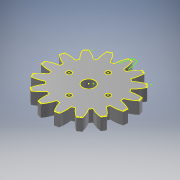
# Autodesk Inventor part: Spur Gear1
Saved by Autodesk Inventor 2017 (Build 210142000, 142)
## iProperties
Created: 2018-10-15
Part Number: Spur Gear1
Material: Steel
Document SubType Name: Modeling
Designer: Tom
Categories: <?xml version="1.0" encoding="UTF-16"?> <MemberInstance><Categories><FamilyTemplate><FamilyTemplateParameter ValueType="xs:double" Id="1" ObjectReferenceKey="da_z" ObjectType="kUserParameterObject"/><FamilyTemplateParameter ValueType="xs:double" Id="2" ObjectReferenceKey="da_b" ObjectType="kUserParameterObject"/><FamilyTemplateParameter ValueType="xs:double" Id="3" ObjectReferenceKey="da_beta" ObjectType="kUserParameterObject"/><FamilyTemplateParameter ValueType="xs:double" Id="4" ObjectReferenceKey="da_da" ObjectType="kUserParameterObject"/><FamilyTemplateParameter ValueType="xs:double" Id="5" ObjectReferenceKey="da_aw" ObjectType="kUserParameterObject"/><FamilyTemplateParameter ValueType="xs:string" Id="6" ObjectReferenceKey="EAIAABAAAACIAQAAAAAAAIAAAAAAAAAA" ObjectType="83910656" SubObjectId="SurfaceGeometry"/></FamilyTemplate><ParamToTemplateMap><ParamToTemplate CategoryParameter="//CategoryParameter[@InternalName='046C89C9-8512-4d59-83FE-43B91F4F132A']" TemplateParameter="1"/><ParamToTemplate CategoryParameter="//CategoryParameter[@InternalName='2552DF32-E462-4b46-AEBF-C6C7768E72AC']" TemplateParameter="2"/><ParamToTemplate CategoryParameter="//CategoryParameter[@InternalName='C9EE641D-15FC-4fae-A226-E94C4372FDD7']" TemplateParameter="3"/><ParamToTemplate><ParamToTemplate CategoryParameter="//CategoryParameter[@InternalName='00B6519A-459B-49c7-AD84-2E56D39A5744']" ConstantValue="0.000000"/></ParamToTemplate><ParamToTemplate><ParamToTemplate CategoryParameter="//CategoryParameter[@InternalName='04B31F0E-C7A6-4894-AA32-9629BEFACF47']" ConstantValue="1.000000"/></ParamToTemplate><ParamToTemplate><ParamToTemplate CategoryParameter="//CategoryParameter[@InternalName='43CBEC2E-7847-49e7-A936-2F7889FCB2D9']" ConstantValue="0.250000"/></ParamToTemplate><ParamToTemplate><ParamToTemplate CategoryParameter="//CategoryParameter[@InternalName='B1EFC894-105D-4ebd-86BF-FA20ED196853']" ConstantValue="0.350000"/></ParamToTemplate><ParamToTemplate><ParamToTemplate CategoryParameter="//CategoryParameter[@InternalName='51175063-3D10-4879-93E8-6246FE8B403D']" ConstantValue="2060000000.000000"/></ParamToTemplate><ParamToTemplate><ParamToTemplate CategoryParameter="//CategoryParameter[@InternalName='A3A52E27-4454-46a9-B0BD-C932399B70AF']" ConstantValue="0.300000"/></ParamToTemplate><ParamToTemplate><ParamToTemplate CategoryParameter="//CategoryParameter[@InternalName='91B76062-C214-41d9-B1B9-14D2AB99603D']" ConstantValue="0.200000"/></ParamToTemplate><ParamToTemplate><ParamToTemplate CategoryParameter="//CategoryParameter[@InternalName='374E806E-8B8A-4dda-A9AA-1039D6500AD2']" ConstantValue="5.000000"/></ParamToTemplate><ParamToTemplate><ParamToTemplate CategoryParameter="//CategoryParameter[@InternalName='2D373A89-B862-43d6-8D0B-0CBF12AB9F6C']" ConstantValue="0.349066"/></ParamToTemplate><ParamToTemplate CategoryParameter="//CategoryParameter[@InternalName='37777632-D6A2-4fac-9D53-DB8ACD95C989']" TemplateParameter="4"/><ParamToTemplate CategoryParameter="//CategoryParameter[@InternalName='FD1017F1-B727-4f7e-9707-0F86F1FF9423']" TemplateParameter="5"/><ParamToTemplate><ParamToTemplate CategoryParameter="//CategoryParameter[@InternalName='9E1B4470-B2D3-4ff1-B813-535BB4CDF51A']" ConstantValue="3520000.000000"/></ParamToTemplate><ParamToTemplate><ParamToTemplate CategoryParameter="//CategoryParameter[@InternalName='F8452263-BFF6-458c-9FB1-07C4B99E95CD']" ConstantValue="11400000.000000"/></ParamToTemplate><ParamToTemplate><ParamToTemplate CategoryParameter="//CategoryParameter[@InternalName='3E3BB259-FD49-497f-8171-6EBC954A3479']" ConstantValue="2.000000"/></ParamToTemplate><ParamToTemplate CategoryParameter="//CategoryParameter[@InternalName='27C3BAF2-7550-4e4b-AE2C-0DB134B7D9B7']" TemplateParameter="6"/></ParamToTemplateMap><Category DisplayName="Gear" InternalName="DC85795E-93AB-48d5-8EEE-5A27447B64BD" Mnemonic="Gear"><CategoryParameter DisplayName="z" InternalName="046C89C9-8512-4d59-83FE-43B91F4F132A" Mnemonic="z"/><CategoryParameter DisplayName="b" InternalName="2552DF32-E462-4b46-AEBF-C6C7768E72AC" Mnemonic="b"/><CategoryParameter DisplayName="||b|" InternalName="C9EE641D-15FC-4fae-A226-E94C4372FDD7" Mnemonic="beta"/><CategoryParameter DisplayName="x" InternalName="00B6519A-459B-49c7-AD84-2E56D39A5744" Mnemonic="x"/><CategoryParameter DisplayName="a*" InternalName="04B31F0E-C7A6-4894-AA32-9629BEFACF47" Mnemonic="a"/><CategoryParameter DisplayName="c*" InternalName="43CBEC2E-7847-49e7-A936-2F7889FCB2D9" Mnemonic="c"/><CategoryParameter DisplayName="r|.f|*" InternalName="B1EFC894-105D-4ebd-86BF-FA20ED196853" Mnemonic="rf"/><CategoryParameter DisplayName="E" InternalName="51175063-3D10-4879-93E8-6246FE8B403D" Mnemonic="E"/><CategoryParameter DisplayName="||m|" InternalName="A3A52E27-4454-46a9-B0BD-C932399B70AF" Mnemonic="mi"/><Category DisplayName="SpurGear" InternalName="26C5A22E-A91E-4dfd-A3B3-23CCAFAE1764" Mnemonic="SpurGear"><CategoryParameter DisplayName="m" InternalName="91B76062-C214-41d9-B1B9-14D2AB99603D" Mnemonic="m"/><CategoryParameter DisplayName="P" InternalName="374E806E-8B8A-4dda-A9AA-1039D6500AD2" Mnemonic="PP"/><CategoryParameter DisplayName="||a|" InternalName="2D373A89-B862-43d6-8D0B-0CBF12AB9F6C" Mnemonic="alpha"/><CategoryParameter DisplayName="d|.a|" InternalName="37777632-D6A2-4fac-9D53-DB8ACD95C989" Mnemonic="da"/><CategoryParameter DisplayName="a|.w|" InternalName="FD1017F1-B727-4f7e-9707-0F86F1FF9423" Mnemonic="aw"/><CategoryParameter DisplayName="||s||.Flim|" InternalName="9E1B4470-B2D3-4ff1-B813-535BB4CDF51A" Mnemonic="sFlim"/><CategoryParameter DisplayName="||s||.Hlim|" InternalName="F8452263-BFF6-458c-9FB1-07C4B99E95CD" Mnemonic="sHlim"/><CategoryParameter DisplayName="type" InternalName="3E3BB259-FD49-497f-8171-6EBC954A3479" Mnemonic="type"/><CategoryParameter DisplayName="PitchDiameter" InternalName="27C3BAF2-7550-4e4b-AE2C-0DB134B7D9B7" Mnemonic="IDS_PITCHDIAM"/></Category></Category></Categories></MemberInstance>
Density: 1 g/cm^3
Appearance: Steel
CustomPartVersion: 1
Author: Tom
Autodesk Inventor part; units mm, degrees
sketch "Sketch1" plane through (0, 0, 0) normal (0, 0, 1) x (1, 0, 0)
  circle A0 centre (0, 0) radius 17
  dimension "d0" = 34
  constraints: 1 centre point
  measures "d0" diameter of A0
extrude "Extrusion1" add sketch "Sketch1" along normal blind 5
ref_plane "Work Plane2" through (0, 0, 2.5) normal (0, 0, 1) x (1, 0, 0)
sketch "Sketch2" plane through (0, 0, 0) normal (0, 0, -1) x (-1, 0, 0)
  circle A0 centre (0, 0) radius 17 projected
  circle A1 centre (0, 0) radius 15
  dimension "d3" = 30
  constraints: 1 centre point, 1 coincident
  measures "d3" diameter of A1
surface extrude "Pitch Diameter" sketch "Sketch2" against normal through all shown no curves A1
ref_plane "Work Plane8" through (0, 0, 0) normal (0.9781476, 0.2079117, 0) x (0, 0, 1)
ref_plane "Work Plane9" through (0, 0, 0) normal (1, 0, 0) x (0, 1, 0)
spur gear teeth "Spur Gear" teeth 15 pitch diameter 30 tip diameter 34 root diameter 25 face width 5 start plane through (0, 0, 0) normal (0, 0, -1) x (-1, 0, 0)
sketch "Sketch3" plane through (0, 0, 5) normal (0, 0, 1) x (1, 0, 0)
  arc A0 (-6.0923, 15.8709) -> (-7.7178, 15.1471) centre (0, 0) ccw projected
  circle A1 centre (0, 0) radius 8
  point P0 (0, 8)
  point P1 (8, 0)
  point P2 (0, -8)
  point P3 (-8, 0)
  dimension "d49" = 16
  constraints: 4 point on circle, 1 centre point, 1 coincident
  measures "d49" diameter of A1
hole "Hole1" at (0, 8, 5) at (8, 0, 5) at (0, -8, 5) at (-8, 0, 5) direction (0, 0, -1) diameter 2 end through all
sketch "Sketch4" plane through (0, 0, 5) normal (0, 0, 1) x (1, 0, 0)
  arc A0 (-6.0923, 15.8709) -> (-7.7178, 15.1471) centre (0, 0) ccw projected
  constraints: 1 coincident
hole "Hole2" at (0, 0, 5) direction (0, 0, -1) diameter 5 end through all
sketch "Sketch5" plane through (0, 0, 5) normal (0, 0, 1) x (1, 0, 0)
  circle A0 centre (0, 0) radius 2.5 projected
  circle A1 centre (0, -8) radius 1 projected
  circle A2 centre (0, 8) radius 1 projected
  circle A3 centre (8, 0) radius 1 projected
  circle A4 centre (-8, 0) radius 1 projected
  arc A5 (-7.7178, 15.1471) -> (-6.808, 10.4834) centre (6.4313, 15.4869) ccw projected
  arc A6 (-6.808, 10.4834) -> (-7.8665, 9.7143) centre (0, 0) ccw projected
  arc A7 (-7.8665, 9.7143) -> (-12.0208, 12.0208) centre (-16.7163, -1.3309) ccw projected
  arc A8 (-12.0208, 12.0208) -> (-13.2115, 10.6984) centre (0, 0) ccw projected
  arc A9 (-13.2115, 10.6984) -> (-10.4834, 6.808) centre (-0.4238, 16.7638) ccw projected
  arc A10 (-10.4834, 6.808) -> (-11.1376, 5.6749) centre (0, 0) ccw projected
  arc A11 (-11.1376, 5.6749) -> (-15.8709, 6.0923) centre (-14.7298, -8.0149) ccw projected
  arc A12 (-15.8709, 6.0923) -> (-16.4207, 4.3999) centre (0, 0) ccw projected
  arc A13 (-16.4207, 4.3999) -> (-12.3461, 1.9554) centre (-7.2056, 15.1422) ccw projected
  arc A14 (-12.3461, 1.9554) -> (-12.4829, 0.6542) centre (0, 0) ccw projected
  arc A15 (-12.4829, 0.6542) -> (-16.9767, -0.8897) centre (-10.1964, -13.3131) ccw projected
  arc A16 (-16.9767, -0.8897) -> (-16.7907, -2.6594) centre (0, 0) ccw projected
  arc A17 (-16.7907, -2.6594) -> (-12.0741, -3.2352) centre (-12.7415, 10.9023) ccw projected
  arc A18 (-12.0741, -3.2352) -> (-11.6698, -4.4796) centre (0, 0) ccw projected
  arc A19 (-11.6698, -4.4796) -> (-15.1471, -7.7178) centre (-3.8999, -16.3094) ccw projected
  arc A20 (-15.1471, -7.7178) -> (-14.2574, -9.2589) centre (0, 0) ccw projected
  arc A21 (-14.2574, -9.2589) -> (-9.7143, -7.8665) centre (-16.0743, 4.7773) ccw projected
  arc A22 (-9.7143, -7.8665) -> (-8.8388, -8.8388) centre (0, 0) ccw projected
  arc A23 (-8.8388, -8.8388) -> (-10.6984, -13.2115) centre (3.0709, -16.4856) ccw projected
  arc A24 (-10.6984, -13.2115) -> (-9.2589, -14.2574) centre (0, 0) ccw projected
  arc A25 (-9.2589, -14.2574) -> (-5.6749, -11.1376) centre (-16.6277, -2.1737) ccw projected
  arc A26 (-5.6749, -11.1376) -> (-4.4796, -11.6698) centre (0, 0) ccw projected
  arc A27 (-4.4796, -11.6698) -> (-4.3999, -16.4207) centre (9.5107, -13.8113) ccw projected
  arc A28 (-4.3999, -16.4207) -> (-2.6594, -16.7907) centre (0, 0) ccw projected
  arc A29 (-2.6594, -16.7907) -> (-0.6542, -12.4829) centre (-14.306, -8.7489) ccw projected
  arc A30 (-0.6542, -12.4829) -> (0.6542, -12.4829) centre (0, 0) ccw projected
  arc A31 (0.6542, -12.4829) -> (2.6594, -16.7907) centre (14.306, -8.7489) ccw projected
  arc A32 (2.6594, -16.7907) -> (4.3999, -16.4207) centre (0, 0) ccw projected
  arc A33 (4.3999, -16.4207) -> (4.4796, -11.6698) centre (-9.5107, -13.8113) ccw projected
  arc A34 (4.4796, -11.6698) -> (5.6749, -11.1376) centre (0, 0) ccw projected
  arc A35 (5.6749, -11.1376) -> (9.2589, -14.2574) centre (16.6277, -2.1737) ccw projected
  arc A36 (9.2589, -14.2574) -> (10.6984, -13.2115) centre (0, 0) ccw projected
  arc A37 (10.6984, -13.2115) -> (8.8388, -8.8388) centre (-3.0709, -16.4856) ccw projected
  arc A38 (8.8388, -8.8388) -> (9.7143, -7.8665) centre (0, 0) ccw projected
  arc A39 (9.7143, -7.8665) -> (14.2574, -9.2589) centre (16.0743, 4.7773) ccw projected
  arc A40 (14.2574, -9.2589) -> (15.1471, -7.7178) centre (0, 0) ccw projected
  arc A41 (15.1471, -7.7178) -> (11.6698, -4.4796) centre (3.8999, -16.3094) ccw projected
  arc A42 (11.6698, -4.4796) -> (12.0741, -3.2352) centre (0, 0) ccw projected
  arc A43 (12.0741, -3.2352) -> (16.7907, -2.6594) centre (12.7415, 10.9023) ccw projected
  arc A44 (16.7907, -2.6594) -> (16.9767, -0.8897) centre (0, 0) ccw projected
  arc A45 (16.9767, -0.8897) -> (12.4829, 0.6542) centre (10.1964, -13.3131) ccw projected
  arc A46 (12.4829, 0.6542) -> (12.3461, 1.9554) centre (0, 0) ccw projected
  arc A47 (12.3461, 1.9554) -> (16.4207, 4.3999) centre (7.2056, 15.1422) ccw projected
  arc A48 (16.4207, 4.3999) -> (15.8709, 6.0923) centre (0, 0) ccw projected
  arc A49 (15.8709, 6.0923) -> (11.1376, 5.6749) centre (14.7298, -8.0149) ccw projected
  arc A50 (11.1376, 5.6749) -> (10.4834, 6.808) centre (0, 0) ccw projected
  arc A51 (10.4834, 6.808) -> (13.2115, 10.6984) centre (0.4238, 16.7638) ccw projected
  arc A52 (13.2115, 10.6984) -> (12.0208, 12.0208) centre (0, 0) ccw projected
  arc A53 (12.0208, 12.0208) -> (7.8665, 9.7143) centre (16.7163, -1.3309) ccw projected
  arc A54 (7.8665, 9.7143) -> (6.808, 10.4834) centre (0, 0) ccw projected
  arc A55 (6.808, 10.4834) -> (7.7178, 15.1471) centre (-6.4313, 15.4869) ccw projected
  arc A56 (7.7178, 15.1471) -> (6.0923, 15.8709) centre (0, 0) ccw projected
  arc A57 (6.0923, 15.8709) -> (3.2352, 12.0741) centre (15.8124, 5.5833) ccw projected
  arc A58 (3.2352, 12.0741) -> (1.9554, 12.3461) centre (0, 0) ccw projected
  arc A59 (1.9554, 12.3461) -> (0.8897, 16.9767) centre (-12.1744, 11.5321) ccw projected
  arc A60 (0.8897, 16.9767) -> (-0.8897, 16.9767) centre (0, 0) ccw projected
  arc A61 (-0.8897, 16.9767) -> (-1.9554, 12.3461) centre (12.1744, 11.5321) ccw projected
  arc A62 (-1.9554, 12.3461) -> (-3.2352, 12.0741) centre (0, 0) ccw projected
  arc A63 (-3.2352, 12.0741) -> (-6.0923, 15.8709) centre (-15.8124, 5.5833) ccw projected
  arc A64 (-6.0923, 15.8709) -> (-7.7178, 15.1471) centre (0, 0) ccw projected
  arc A65 (2.9554, 13.3461) -> (1.8897, 17.9767) centre (-11.1744, 12.5321) ccw
  arc A66 (1.8897, 17.9767) -> (0.1103, 17.9767) centre (1, 1) ccw
  arc A67 (0.1103, 17.9767) -> (-0.9554, 13.3461) centre (13.1744, 12.5321) ccw
  constraints: 6 point on circle, 3 centre point
sketch "Sketch6" plane through (0, 0, 0) normal (0, 0, 1) x (1, 0, 0)
  arc A0 (3.9109, 0) -> (2.8451, 4.6306) centre (-10.219, -0.814) ccw
  arc A1 (2.8451, 4.6306) -> (1.0657, 4.6306) centre (1.9554, -12.3461) ccw
  arc A2 (1.0657, 4.6306) -> (0, 0) centre (14.1298, -0.814) ccw
  point P0 (0, 0)
  constraints: 6 point on circle, 3 centre point
equation "\"d0\" = da_da"
equation "\"d1\" = da_b"
equation "\"d3\" = da_dw"
equation "\"d16\" = da_aw"
equation "\"d43\" = da_aw"
equation "\"d46\" = da_aw"
equation "\"da_da\" = 34"
equation "\"da_b\" = 5"
equation "\"da_dw\" = 30"
equation "\"da_aw\" = 72"
body "Solid1"
body "Srf1"
